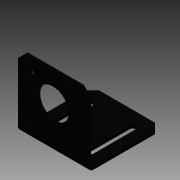
# Autodesk Inventor part: Stepper Motor Mount
Saved by Autodesk Inventor 2015 (Build 190159000, 159)
## iProperties
Created: 2015-02-23
Part Number: Stepper Motor Mount
Material: Aluminum 6061
Document SubType Name: Sheet Metal
Designer: Andrew
Density: 2.7 g/cm^3
Sheet Metal Rule: Default_mm
Appearance: Anodized - Black
Author: Andrew
Autodesk Inventor part; units mm, degrees
ref_plane "YZ Plane" through (0, 0, 0) normal (1, 0, 0) x (0, 1, 0)
ref_plane "XZ Plane" through (0, 0, 0) normal (0, 1, 0) x (-1, 0, 0)
ref_plane "XY Plane" through (0, 0, 0) normal (0, 0, 1) x (1, 0, 0)
sketch "Sketch1" plane through (0, 0, 0) normal (0, 0, 1) x (1, 0, 0)
  line L0 (-25, 49) -> (25, 49)
  line L1 (25, 49) -> (25, -51)
  line L2 (25, -51) -> (-25, -51)
  line L3 (-25, -51) -> (-25, 49)
  circle A0 centre (-15.5, 39.5) radius 1.75
  circle A1 centre (15.5, 39.5) radius 1.75
  circle A2 centre (15.5, 8.5) radius 1.75
  circle A3 centre (-15.5, 8.5) radius 1.75
  circle A4 centre (0, 28) radius 11.05
  arc A5 (-12.9, -10) -> (-17.1, -10) centre (-15, -10) ccw
  arc A6 (17.1, -10) -> (12.9, -10) centre (15, -10) ccw
  arc A7 (-17.1, -40) -> (-12.9, -40) centre (-15, -40) ccw
  arc A8 (12.9, -40) -> (17.1, -40) centre (15, -40) ccw
  line L4 (0, 69) -> (0, -71) projected
  line L5 (-35, 0) -> (35, 0) projected
  line L6 (-12.9, -40) -> (-12.9, -10)
  line L7 (-17.1, -10) -> (-17.1, -40)
  line L8 (12.9, -40) -> (12.9, -10)
  line L9 (17.1, -10) -> (17.1, -40)
  line L10 (-25, 0) -> (25, 0)
  point P0 (0, 0)
  dimension "d0" = 31
  dimension "d1" = 50
  dimension "d2" = 100
  dimension "d3" = 21
  dimension "d4" = 22.1
  dimension "d5" = 49
  dimension "d6" = 31
  dimension "d7" = 3.5
  dimension "d8" = 30
  dimension "d9" = 4.2
  dimension "d10" = 30
  dimension "d11" = 11
  dimension "d12" = 9.5
  dimension "d13" = 9.5
  dimension "d14" = 31
  constraints: 18 end point, 9 centre point, 8 point on circle, 7 tangent, 5 point on line, 4 parallel, 2 equal radius, 1 horizontal, 1 perpendicular, 5 other
  measures "d0" distance of A1.centre A0.centre
  measures "d1" distance between parallel lines of L3 L1
  measures "d2" distance between parallel lines of L2 L0
  measures "d3" distance from line of L0 A4.centre
  measures "d4" diameter of A4
  measures "d5" distance between parallel lines of L5 L0
  measures "d6" distance of A2.centre A1.centre
  measures "d7" diameter of A1
  measures "d8" distance of A7.centre A8.centre
  measures "d9" distance between parallel lines of L7 L6
  measures "d10" distance of A8.centre A6.centre
  measures "d11" distance from line of L2 A8.centre
  measures "d12" distance from line of L0 A1.centre
  measures "d13" distance from line of L1 A1.centre
  measures "d14" distance of A3.centre A2.centre
extrude "Plate1" add sketch "Sketch1" along normal blind 2 contours L0 L4 A4 L5 L3 | L0 L1 L5 L4 A4 | L5 L4 L2 L3 | L5 L1 L2 L4
fold "Fold1" angle 90 bend radius 2 thickness 2 k factor 0.44 line from (-25, 0, 0) to (25, 0, 0) line at bend centre moving side (0, -1, 0) folds toward (0, 0, -1)
chamfer "Corner Chamfer1" distance 5 angle 45 4 edges at (-25, 49, 1) (25, 49, 1) (-25, -0.7381, -50.7381) (25, -0.7381, -50.7381)
equation "\"d12\" = d13"
equation "\"d16\" = BendReliefWidth"
equation "\"d17\" = BendReliefDepth"
equation "\"d18\" = MinimumRemnant"
equation "\"d19\" = BendRadius"
equation "\"d21\" = BendRadius"
equation "\"BendRadius\" = Thickness"
equation "\"BendReliefWidth\" = Thickness"
equation "\"BendReliefDepth\" = 0.5 * Thickness"
equation "\"CornerReliefSize\" = 4 * Thickness"
equation "\"MinimumRemnant\" = 2 * Thickness"
equation "\"TransitionRadius\" = BendRadius"
equation "\"JacobiRadiusSize\" = BendRadius"
equation "\"GapSize\" = Thickness"
equation "\"d15\" = BendRadius"
equation "\"Thickness\" = 2"
body "Solid1"
